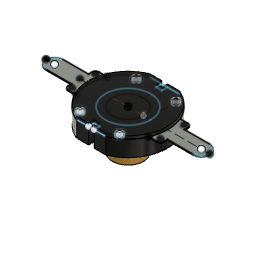
button mxuteuk YX-1214 (Autodesk Fusion 360 design; units mm, degrees)
Autodesk Fusion 360 part; units mm, degrees
sketch "Sketch1" plane through (0, 0, 0) normal (0, 0, 1) x (1, 0, 0)
  line L0 (0, 6.5) -> (2.5978, 6.5)
  line L1 (2.5978, 6.5) -> (-2.5981, 6.5)
  line L2 (0, -6.5) -> (2.5978, -6.5)
  line L3 (0, -6.5) -> (-2.5981, -6.5)
  arc A0 (2.5978, -6.5) -> (2.5978, 6.5) centre (0, 0) ccw
  arc A1 (-2.5981, 6.5) -> (-2.5981, -6.5) centre (0, 0) ccw
  circle A2 centre (0, 0) radius 4
  circle A3 centre (0, 0) radius 2.75
  line L4 (0, 6.5) -> (-0.5, 6.5) construction
  line L5 (-0.5, 5.5) -> (-0.5, 6.5)
  line L6 (0.5, 5.5) -> (0.5, 6.5)
  line L7 (0.5, 5.5) -> (-0.5, 5.5)
  line L8 (2.75, 0) -> (-2.75, 0) construction
  line L9 (-0.5, -5.5) -> (-0.5, -6.5)
  line L10 (0.5, -5.5) -> (-0.5, -5.5)
  line L11 (0.5, -5.5) -> (0.5, -6.5)
  line L12 (0, 0) -> (0, 5.5) construction
  line L13 (0, 0) -> (3.5, 0) construction
  line L14 (3.5, 0) -> (3.5, 5) construction
  circle A4 centre (3.5, 5) radius 0.65
  line L15 (3.5, 5) -> (3.5, 5.4)
  arc A5 (3.6411, 5.4) -> (3.38, 5.4) centre (3.5105, 5.4093) ccw
  line L16 (3.5, 5) -> (4.15, 5) construction
  arc A6 (3.38, 4.6) -> (3.6411, 4.6) centre (3.5105, 4.5907) ccw
  arc A7 (3.1018, 5.1323) -> (3.1018, 4.8712) centre (3.0925, 5.0018) ccw
  arc A8 (3.9018, 4.8712) -> (3.9018, 5.1323) centre (3.9111, 5.0018) ccw
  line L17 (3.9018, 5.1323) -> (3.6411, 5.1323)
  line L18 (3.9018, 4.8712) -> (3.6411, 4.8712)
  line L19 (3.1018, 5.1323) -> (3.38, 5.1323)
  line L20 (3.1018, 4.8712) -> (3.38, 4.8712)
  line L21 (3.38, 5.1323) -> (3.38, 5.4)
  line L22 (3.6411, 5.1323) -> (3.6411, 5.4)
  line L23 (3.38, 4.8712) -> (3.38, 4.6)
  line L24 (3.6411, 4.8712) -> (3.6411, 4.6)
  arc A9 (-3.38, 5.4) -> (-3.6411, 5.4) centre (-3.5105, 5.4093) ccw
  line L25 (-3.6411, 5.1323) -> (-3.6411, 5.4)
  line L26 (-3.9018, 5.1323) -> (-3.6411, 5.1323)
  arc A10 (-3.9018, 5.1323) -> (-3.9018, 4.8712) centre (-3.9111, 5.0018) ccw
  line L27 (-3.9018, 4.8712) -> (-3.6411, 4.8712)
  line L28 (-3.6411, 4.8712) -> (-3.6411, 4.6)
  arc A11 (-3.6411, 4.6) -> (-3.38, 4.6) centre (-3.5105, 4.5907) ccw
  line L29 (-3.38, 4.8712) -> (-3.38, 4.6)
  line L30 (-3.1018, 4.8712) -> (-3.38, 4.8712)
  arc A12 (-3.1018, 4.8712) -> (-3.1018, 5.1323) centre (-3.0925, 5.0018) ccw
  line L31 (-3.1018, 5.1323) -> (-3.38, 5.1323)
  line L32 (-3.38, 5.1323) -> (-3.38, 5.4)
  circle A13 centre (-3.5, 5) radius 0.65
  arc A14 (-3.38, -4.6) -> (-3.6411, -4.6) centre (-3.5105, -4.5907) ccw
  line L33 (-3.6411, -4.8712) -> (-3.6411, -4.6)
  line L34 (-3.9018, -4.8712) -> (-3.6411, -4.8712)
  arc A15 (-3.9018, -4.8712) -> (-3.9018, -5.1323) centre (-3.9111, -5.0018) ccw
  line L35 (-3.9018, -5.1323) -> (-3.6411, -5.1323)
  line L36 (-3.6411, -5.1323) -> (-3.6411, -5.4)
  arc A16 (-3.6411, -5.4) -> (-3.38, -5.4) centre (-3.5105, -5.4093) ccw
  line L37 (-3.38, -5.1323) -> (-3.38, -5.4)
  line L38 (-3.1018, -5.1323) -> (-3.38, -5.1323)
  arc A17 (-3.1018, -5.1323) -> (-3.1018, -4.8712) centre (-3.0925, -5.0018) ccw
  line L39 (-3.1018, -4.8712) -> (-3.38, -4.8712)
  line L40 (-3.38, -4.8712) -> (-3.38, -4.6)
  circle A18 centre (-3.5, -5) radius 0.65
  arc A19 (3.38, -5.4) -> (3.6411, -5.4) centre (3.5105, -5.4093) ccw
  line L41 (3.6411, -5.1323) -> (3.6411, -5.4)
  line L42 (3.9018, -5.1323) -> (3.6411, -5.1323)
  arc A20 (3.9018, -5.1323) -> (3.9018, -4.8712) centre (3.9111, -5.0018) ccw
  line L43 (3.9018, -4.8712) -> (3.6411, -4.8712)
  line L44 (3.6411, -4.8712) -> (3.6411, -4.6)
  arc A21 (3.6411, -4.6) -> (3.38, -4.6) centre (3.5105, -4.5907) ccw
  line L45 (3.38, -4.8712) -> (3.38, -4.6)
  line L46 (3.1018, -4.8712) -> (3.38, -4.8712)
  arc A22 (3.1018, -4.8712) -> (3.1018, -5.1323) centre (3.0925, -5.0018) ccw
  line L47 (3.38, -5.1323) -> (3.38, -5.4)
  line L48 (3.1018, -5.1323) -> (3.38, -5.1323)
  circle A23 centre (3.5, -5) radius 0.65
  line L49 (-7, 0) -> (-8.5, 0) construction
  arc A24 (8.5, 2.0828) -> (7.8349, 2.75) centre (7.8327, 2.0828) ccw
  line L50 (7.8349, 2.75) -> (6.4371, 2.75)
  arc A25 (14.4999, -0.017) -> (13.0058, 1.5) centre (13.0058, 0.0057) ccw
  arc A26 (14.4999, -0.017) -> (13.0058, 1.5) centre (13.0058, 0.0057) ccw construction
  circle A27 centre (13, 0) radius 0.5
  line L51 (8.5, 2.0828) -> (8.5, 1.5)
  line L52 (13.0058, 1.5) -> (8.5, 1.5)
  line L53 (14.4999, -0.017) -> (6.9999, 0) construction
  line L54 (12.9989, -1.5271) -> (8.4932, -1.5068)
  arc A28 (7.8225, -2.7537) -> (8.4906, -2.0895) centre (7.8233, -2.0865) ccw
  line L55 (7.8225, -2.7537) -> (6.4247, -2.7474)
  arc A29 (12.9989, -1.5271) -> (14.4999, -0.017) centre (13.0057, -0.0328) ccw
  line L56 (8.4906, -2.0895) -> (8.4932, -1.5068)
  arc A30 (-13.0058, 1.5) -> (-14.4999, -0.017) centre (-13.0058, 0.0057) ccw
  line L57 (-13.0058, 1.5) -> (-8.5, 1.5)
  line L58 (-8.5, 2.0828) -> (-8.5, 1.5)
  arc A31 (-7.8349, 2.75) -> (-8.5, 2.0828) centre (-7.8327, 2.0828) ccw
  line L59 (-7.8349, 2.75) -> (-6.4371, 2.75)
  arc A32 (-14.4999, -0.017) -> (-12.9989, -1.5271) centre (-13.0057, -0.0328) ccw
  line L60 (-8.4906, -2.0895) -> (-8.4932, -1.5068)
  arc A33 (-8.4906, -2.0895) -> (-7.8225, -2.7537) centre (-7.8233, -2.0865) ccw
  line L61 (-7.8225, -2.7537) -> (-6.4247, -2.7474)
  line L62 (-12.9989, -1.5271) -> (-8.4932, -1.5068)
  circle A34 centre (-13, 0) radius 0.5
  dimension "d10" = 5.5
  dimension "d11" = 3.5
  dimension "d12" = 5
  dimension "d13" = 1.3
  dimension "d14" = 1.5
  dimension "d19" = 1
  dimension "d20" = 7.5
  dimension "d21" = 0.259
  constraint parallel L0 L1
  constraint coincident A0.centre A1.centre
  constraint concentric A0 A2
  constraint concentric A1 A3
  constraint parallel L1 L4
  constraint coincident L0 L6.end
  constraint coincident A3 L8.start
  constraint coincident A3 L8.end
  constraint symmetric L4.end L8 L9.end
  constraint symmetric L6.start L8 L10.start
  constraint symmetric L5.start L8 L9.start
  constraint symmetric L6.end L8 L11.end
  constraint midpoint L7 L12.end
  constraint perpendicular L12 L13
  constraint perpendicular L13 L14
  constraint coincident L14.end A4.centre
  constraint parallel L14 L15
  constraint coincident A4 L16.end
  constraint perpendicular L15 L16
  constraint symmetric A5.start L16 A6.end
  constraint symmetric A5.end L16 A6.start
  constraint symmetric A5 L16 A6
  constraint perpendicular L19 L21
  constraint perpendicular L17 L22
  constraint perpendicular L20 L23
  constraint perpendicular L18 L24
  constraint symmetric L12 A4 A13
  constraint symmetric L12 A5.start A9.end
  constraint symmetric L12 A5.end A9.start
  constraint symmetric L12 A5 A9
  constraint symmetric L12 A6.end L28.end
  constraint symmetric L12 A6.start A11.end
  constraint symmetric L12 A6 A11
  constraint symmetric L12 A8.start A10.end
  constraint symmetric L12 A8.end L26.start
  constraint symmetric L12 A7.end L30.start
  constraint symmetric L12 A7.start A12.end
  constraint symmetric L12 A7 A12
  constraint symmetric L12 A8 A10
  constraint symmetric L12 L17.end L25.start
  constraint symmetric L12 L18.end L27.end
  constraint symmetric L12 L19.end L31.end
  constraint symmetric L12 L20.end L29.start
  constraint symmetric L8 A4 A23
  constraint symmetric L8 A5.start A19.end
  constraint symmetric L8 A5.end A19.start
  constraint symmetric L8 A5 A19
  constraint symmetric L8 A6.end L44.end
  constraint symmetric L8 A6.start A21.end
  constraint symmetric L8 A6 A21
  constraint symmetric L8 A8.start A20.end
  constraint symmetric L8 A8.end L42.start
  constraint symmetric L8 A7.end L46.start
  constraint symmetric L8 A7.start A22.end
  constraint symmetric L8 A7 A22
  constraint symmetric L8 A8 A20
  constraint symmetric L8 L17.end L41.start
  constraint symmetric L8 L18.end L43.end
  constraint symmetric L8 L19.end L47.start
  constraint symmetric L8 L20.end L45.start
  constraint symmetric L8 A9.end L36.end
  constraint symmetric L8 A9.start A16.end
  constraint symmetric L8 A9 A16
  constraint symmetric L8 L25.start L35.end
  constraint symmetric L8 L26.start A15.end
  constraint symmetric L8 A10.end L34.start
  constraint symmetric L8 A10 A15
  constraint symmetric L8 L27.end L33.start
  constraint symmetric L8 L28.end A14.end
  constraint symmetric L8 A11.end A14.start
  constraint symmetric L8 A11 A14
  constraint symmetric L8 L29.start L39.end
  constraint symmetric L8 L30.start A17.end
  constraint symmetric L8 A12.end L38.start
  constraint symmetric L8 A12 A17
  constraint symmetric L8 L31.end L37.start
  constraint symmetric L8 A13 A18
  constraint midpoint A1 L49.start
  constraint horizontal L49
  constraint coincident A0 L50.end
  constraint horizontal L50
  constraint tangent A24 L51
  constraint vertical L51
  constraint midpoint A0 L53.end
  constraint symmetric A24.end L53 A28.start
  constraint symmetric A24.start L53 A28.end
  constraint symmetric A24 L53 A28
  constraint symmetric L50.end L53 L55.end
  constraint symmetric A25.end L53 L54.start
  constraint symmetric A25.start L53 A26.start
  constraint symmetric A26 L53 A29
  constraint symmetric L51.end L53 L54.end
  constraint symmetric L12 A24.end A31.start
  constraint symmetric L12 A24.start L58.start
  constraint symmetric L12 A24 A31
  constraint symmetric L12 L50.end L59.end
  constraint symmetric L12 A25.end A30.start
  constraint symmetric L12 A25.start A30.end
  constraint symmetric L12 A25 A30
  constraint symmetric L12 A27 A34
  constraint symmetric L12 L51.end L57.end
  constraint symmetric L12 L54.start A32.end
  constraint symmetric L12 L54.end L60.end
  constraint symmetric L12 A28.end L60.start
  constraint symmetric L12 A28.start A33.end
  constraint symmetric L12 A28 A33
  constraint symmetric L12 L55.end L61.end
  constraint symmetric L12 A29 A32
  measures "d10" distance of L8.start L8.end
  measures "d11" distance of A0.centre L13.end
  measures "d12" distance of L13.end L14.end
  measures "d13" diameter of A4
  measures "d14" distance of L49.start L49.end
  measures "d19" diameter of A27
  measures "d20" horizontal distance of A25.start L53.end
  measures "d21" angle of L52 L54
extrude "Extrude1" add sketch "Sketch1" against normal blind 0.15 contours A0 A24 L50 A25 L51 L52 L54 A28 L55 A29 L56 | A1 A30 L57 L58 A31 L59 A32 L60 A33 L61 L62 makes body 1 at (-9.8311, -0.0023, 0) makes body 2 at (9.8311, -0.0023, 0)
extrude "Extrude2" add sketch "Sketch1" along normal blind 0.5 and the other way blind 2.85 separate body contours L0 L1 L2 L3 A0 A1 L5 L6 L7 L9 L10 L11 | A4 | A5 A6 A7 A8 L17 L18 L19 L20 L21 L22 L23 L24 | A9 L25 L26 A10 L27 L28 A11 L29 L30 A12 L31 L32 | A13 | A14 L33 L34 A15 L35 L36 A16 L37 L38 A17 L39 L40 | A18 | A19 L41 L42 A20 L43 L44 A21 L45 L46 A22 L47 L48 | A23 makes body 3
extrude "Extrude3" add sketch "Sketch1" along normal blind 0.5 contours A2 | A3 bodies 3
extrude "Extrude4" add sketch "Sketch1" against normal blind 2.8 separate body contours A2 makes body 4
extrude "Extrude5" add 1 faces at (3.5582, -0.3353, -2.8) along direction (0, 0, -1) blind 2 on bodies 4 bodies 4 3
extrude "Extrude6" add sketch "Sketch1" against normal blind 4.8 separate body contours A3 makes body 5
extrude "Extrude7" add 1 faces at (-0.7255, 0.3045, -4.8) along direction (0, 0, -1) blind 2.2 separate body on bodies 5 makes body 6
extrude "Extrude8" cut sketch "Sketch1" along normal blind -2.8 and the other way blind 2.85 contours A4 | A5 A6 A7 A8 L17 L18 L19 L20 L21 L22 L23 L24 | A9 L25 L26 A10 L27 L28 A11 L29 L30 A12 L31 L32 | A13 | A14 L33 L34 A15 L35 L36 A16 L37 L38 A17 L39 L40 | A18 | A19 L41 L42 A20 L43 L44 A21 L45 L46 A22 L47 L48 | A23 bodies 4
combine "Combine1" operation add target body 5 tool bodies 6
extrude "Extrude9" cut sketch "Sketch1" against normal blind 2.5 contours A3 bodies 5
extrude "Extrude10" cut sketch "Sketch1" along normal blind -2.7 and the other way blind 2.8 contours A5 A6 A7 A8 L17 L18 L19 L20 L21 L22 L23 L24 | A9 L25 L26 A10 L27 L28 A11 L29 L30 A12 L31 L32 | A14 L33 L34 A15 L35 L36 A16 L37 L38 A17 L39 L40 | A19 L41 L42 A20 L43 L44 A21 L45 L46 A22 L47 L48 bodies 4
fillet "Fillet1" radius 0.05 12 edges at (-3.6411, -5.2661, -2.8) (-3.5105, -5.5402, -2.8) (-3.38, -5.2661, -2.8) (-3.2409, -5.1323, -2.8) (-2.9617, -5.0018, -2.8) (-3.2409, -4.8712, -2.8) (-3.38, -4.7356, -2.8) (-3.5105, -4.4598, -2.8) (-3.6411, -4.7356, -2.8) (-3.7714, -4.8712, -2.8) (-4.042, -5.0018, -2.8) (-3.7714, -5.1323, -2.8) on bodies 4
fillet "Fillet2" radius 0.05 24 edges at (-3.7714, 4.8712, -2.8) (-4.042, 5.0018, -2.8) (-3.7714, 5.1323, -2.8) (-3.6411, 5.2661, -2.8) (-3.5105, 5.5402, -2.8) (-3.38, 5.2661, -2.8) (-3.2409, 5.1323, -2.8) (-2.9617, 5.0018, -2.8) (-3.2409, 4.8712, -2.8) (-3.38, 4.7356, -2.8) (-3.5105, 4.4598, -2.8) (-3.6411, 4.7356, -2.8) (3.2409, 4.8712, -2.8) (2.9617, 5.0018, -2.8) (3.2409, 5.1323, -2.8) (3.38, 5.2661, -2.8) (3.5105, 5.5402, -2.8) (3.6411, 5.2661, -2.8) (3.7714, 5.1323, -2.8) (4.042, 5.0018, -2.8) (3.7714, 4.8712, -2.8) (3.6411, 4.7356, -2.8) (3.5105, 4.4598, -2.8) (3.38, 4.7356, -2.8) on bodies 4
fillet "Fillet3" radius 0.05 12 edges at (3.2409, -5.1323, -2.8) (2.9617, -5.0018, -2.8) (3.2409, -4.8712, -2.8) (3.38, -4.7356, -2.8) (3.6411, -4.7356, -2.8) (3.5105, -4.4598, -2.8) (3.38, -5.2661, -2.8) (3.5105, -5.5402, -2.8) (3.6411, -5.2661, -2.8) (3.7714, -5.1323, -2.8) (4.042, -5.0018, -2.8) (3.7714, -4.8712, -2.8) on bodies 4
named bodies: "Metal contact L", "Metal contact R", "Body", "yellow button"
